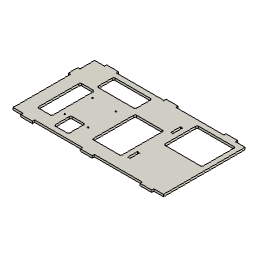
Base Plate (Autodesk Fusion 360 design; units mm, degrees)
Autodesk Fusion 360 part; units mm, degrees
sketch "Sketch1" plane through (0, 0, 0) normal (0, 0, 1) x (1, 0, 0)
  line L0 (160, -90) -> (-160, -90)
  line L1 (-160, -90) -> (-160, 90)
  line L2 (-160, 90) -> (160, 90)
  line L3 (160, 90) -> (160, -90)
  line L4 (160, -90) -> (-160, 90) construction
  line L5 (-160, -90) -> (160, 90) construction
  line L6 (170, 85.5) -> (-180, 85.5) construction
  line L7 (-180, -85.5) -> (170, -85.5) construction
  line L8 (-155.5, 90) -> (-155.5, -90)
  line L9 (-160, 90) -> (-135, 90)
  line L10 (-135, 90) -> (-135, 85.5)
  line L11 (-135, 85.5) -> (-160, 85.5)
  line L12 (-160, 85.5) -> (-160, 90)
  line L13 (-160, -90) -> (-135, -90)
  line L14 (-135, -90) -> (-135, -85.5)
  line L15 (-135, -85.5) -> (-160, -85.5)
  line L16 (-160, -85.5) -> (-160, -90)
  line L17 (-110, -90) -> (-10, -90)
  line L18 (-10, -90) -> (-10, -85.5)
  line L19 (-10, -85.5) -> (-110, -85.5)
  line L20 (-110, -85.5) -> (-110, -90)
  line L21 (-10, -90) -> (15, -90)
  line L22 (15, -90) -> (15, -85.5)
  line L23 (15, -85.5) -> (-10, -85.5)
  line L24 (-10, -85.5) -> (-10, -90)
  line L25 (15, -90) -> (115, -90)
  line L26 (115, -90) -> (115, -85.5)
  line L27 (115, -85.5) -> (15, -85.5)
  line L28 (15, -85.5) -> (15, -90)
  line L29 (115, -90) -> (140, -90)
  line L30 (140, -90) -> (140, -85.5)
  line L31 (140, -85.5) -> (115, -85.5)
  line L32 (115, -85.5) -> (115, -90)
  line L33 (-135, 85.5) -> (-110, 85.5)
  line L34 (-110, 85.5) -> (-110, 90)
  line L35 (-110, 90) -> (-135, 90)
  line L36 (-135, 90) -> (-135, 85.5)
  line L37 (-110, 85.5) -> (-10, 85.5)
  line L38 (-10, 85.5) -> (-10, 90)
  line L39 (-10, 90) -> (-110, 90)
  line L40 (-110, 90) -> (-110, 85.5)
  line L41 (-10, 85.5) -> (15, 85.5)
  line L42 (15, 85.5) -> (15, 90)
  line L43 (15, 90) -> (-10, 90)
  line L44 (-10, 90) -> (-10, 85.5)
  line L45 (15, 85.5) -> (115, 85.5)
  line L46 (115, 85.5) -> (115, 90)
  line L47 (115, 90) -> (15, 90)
  line L48 (15, 90) -> (15, 85.5)
  line L49 (115, 85.5) -> (140, 85.5)
  line L50 (140, 85.5) -> (140, 90)
  line L51 (140, 90) -> (115, 90)
  line L52 (115, 90) -> (115, 85.5)
  line L53 (140, 85.5) -> (160, 85.5)
  line L54 (160, 85.5) -> (160, 90)
  line L55 (160, 90) -> (140, 90)
  line L56 (140, 90) -> (140, 85.5)
  line L57 (140, -90) -> (160, -90)
  line L58 (160, -90) -> (160, -85.5)
  line L59 (160, -85.5) -> (140, -85.5)
  line L60 (140, -85.5) -> (140, -90)
  line L61 (-160, 55) -> (-155.5, 55)
  line L62 (-155.5, 55) -> (-155.5, 35)
  line L63 (-155.5, 35) -> (-160, 35)
  line L64 (-160, 35) -> (-160, 55)
  line L65 (-160, -35) -> (-155.5, -35)
  line L66 (-155.5, -35) -> (-155.5, -55)
  line L67 (-155.5, -55) -> (-160, -55)
  line L68 (-160, -55) -> (-160, -35)
  line L69 (55, 100) -> (55, -100) construction
  line L70 (59.5, 100) -> (59.5, -100) construction
  line L71 (55, 55) -> (59.5, 55)
  line L72 (59.5, 55) -> (59.5, 35)
  line L73 (59.5, 35) -> (55, 35)
  line L74 (55, 35) -> (55, 55)
  line L75 (55, -35) -> (59.5, -35)
  line L76 (59.5, -35) -> (59.5, -55)
  line L77 (59.5, -55) -> (55, -55)
  line L78 (55, -55) -> (55, -35)
  line L79 (-40.5, -43) -> (-89.5, -43) construction
  line L80 (-89.5, -43) -> (-89.5, 15) construction
  line L81 (-89.5, 15) -> (-40.5, 15) construction
  line L82 (-40.5, 15) -> (-40.5, -43) construction
  line L83 (-40.5, -43) -> (-89.5, 15) construction
  line L84 (-89.5, -43) -> (-40.5, 15) construction
  circle A0 centre (-40.5, 15) radius 1.4
  circle A1 centre (-89.5, 15) radius 1.4
  circle A2 centre (-89.5, -43) radius 1.4
  circle A3 centre (-40.5, -43) radius 1.4
  line L85 (-53, -75) -> (-77, -75)
  line L86 (-80, -72) -> (-80, -43)
  line L87 (-77, -40) -> (-53, -40)
  line L88 (-50, -43) -> (-50, -72)
  line L89 (-50, -75) -> (-80, -40) construction
  line L90 (-80, -75) -> (-50, -40) construction
  arc A4 (-77, -40) -> (-80, -43) centre (-77, -43) ccw
  arc A5 (-50, -43) -> (-53, -40) centre (-53, -43) ccw
  arc A6 (-80, -72) -> (-77, -75) centre (-77, -72) ccw
  arc A7 (-53, -75) -> (-50, -72) centre (-53, -72) ccw
  line L91 (-28, 40) -> (-102, 40)
  line L92 (-105, 43) -> (-105, 72)
  line L93 (-102, 75) -> (-28, 75)
  line L94 (-25, 72) -> (-25, 43)
  line L95 (-25, 40) -> (-105, 75) construction
  line L96 (-105, 40) -> (-25, 75) construction
  arc A8 (-102, 75) -> (-105, 72) centre (-102, 72) ccw
  arc A9 (-25, 72) -> (-28, 75) centre (-28, 72) ccw
  arc A10 (-105, 43) -> (-102, 40) centre (-102, 43) ccw
  arc A11 (-28, 40) -> (-25, 43) centre (-28, 43) ccw
  line L97 (147, 5) -> (73, 5)
  line L98 (70, 8) -> (70, 72)
  line L99 (73, 75) -> (147, 75)
  line L100 (150, 72) -> (150, 8)
  line L101 (150, 5) -> (70, 75) construction
  line L102 (70, 5) -> (150, 75) construction
  arc A12 (70, 8) -> (73, 5) centre (73, 8) ccw
  arc A13 (73, 75) -> (70, 72) centre (73, 72) ccw
  arc A14 (150, 72) -> (147, 75) centre (147, 72) ccw
  arc A15 (147, 5) -> (150, 8) centre (147, 8) ccw
  line L103 (42, -60) -> (-12, -60)
  line L104 (-15, -57) -> (-15, 27)
  line L105 (-12, 30) -> (42, 30)
  line L106 (45, 27) -> (45, -57)
  line L107 (45, -60) -> (-15, 30) construction
  line L108 (-15, -60) -> (45, 30) construction
  arc A16 (-12, 30) -> (-15, 27) centre (-12, 27) ccw
  arc A17 (45, 27) -> (42, 30) centre (42, 27) ccw
  arc A18 (-15, -57) -> (-12, -60) centre (-12, -57) ccw
  arc A19 (42, -60) -> (45, -57) centre (42, -57) ccw
  line L109 (-103, -60) -> (-127, -60)
  line L110 (-130, -57) -> (-130, 27)
  line L111 (-127, 30) -> (-103, 30)
  line L112 (-100, 27) -> (-100, -57)
  line L113 (-100, -60) -> (-130, 30) construction
  line L114 (-130, -60) -> (-100, 30) construction
  arc A20 (-127, 30) -> (-130, 27) centre (-127, 27) ccw
  arc A21 (-100, 27) -> (-103, 30) centre (-103, 27) ccw
  arc A22 (-130, -57) -> (-127, -60) centre (-127, -57) ccw
  arc A23 (-103, -60) -> (-100, -57) centre (-103, -57) ccw
  point P0 (-65, -14)
  point P1 (-65, -57.5)
  point P2 (-65, 57.5)
  point P3 (110, 40)
  point P4 (15, -15)
  point P5 (-115, -15)
  dimension "d1" = 320
  dimension "d2" = 180
  dimension "d3" = 4.5
  dimension "d4" = 4.5
  dimension "d5" = 4.5
  dimension "d6" = 25
  dimension "d7" = 25
  dimension "d8" = 100
  dimension "d9" = 25
  dimension "d10" = 25
  dimension "d11" = 100
  dimension "d12" = 25
  dimension "d13" = 25
  dimension "d14" = 100
  dimension "d15" = 25
  dimension "d16" = 100
  dimension "d17" = 25
  dimension "d18" = 20
  dimension "d19" = 20
  dimension "d20" = 35
  dimension "d21" = 35
  dimension "d22" = 215
  dimension "d23" = 4.5
  dimension "d24" = 20
  dimension "d25" = 20
  dimension "d26" = 35
  dimension "d27" = 35
  dimension "d28" = 49
  dimension "d29" = 58
  dimension "d30" = 76
  dimension "d31" = 120
  dimension "d32" = 2.8
  dimension "d33" = 2.8
  dimension "d34" = 2.8
  dimension "d35" = 2.8
  dimension "d46" = 30
  dimension "d47" = 35
  dimension "d48" = 3
  dimension "d49" = 3
  dimension "d50" = 3
  dimension "d51" = 3
  dimension "d52" = 80
  dimension "d53" = 35
  dimension "d54" = 25
  dimension "d55" = 3
  dimension "d56" = 3
  dimension "d57" = 3
  dimension "d58" = 3
  dimension "d65" = 80
  dimension "d66" = 70
  dimension "d67" = 3
  dimension "d68" = 3
  dimension "d69" = 3
  dimension "d70" = 3
  dimension "d71" = 3
  dimension "d72" = 3
  dimension "d73" = 3
  dimension "d74" = 3
  dimension "d75" = 3
  dimension "d76" = 3
  dimension "d77" = 3
  dimension "d78" = 3
  dimension "d103" = 10.5
  dimension "d104" = 10.5
  dimension "d105" = 10.5
  constraint horizontal L0
  constraint perpendicular L0 L1
  constraint parallel L0 L2
  constraint parallel L1 L3
  constraint coincident L4 origin
  constraint coincident L5 origin
  constraint perpendicular L3 L6
  constraint perpendicular L3 L7
  constraint perpendicular L0 L8
  constraint horizontal L9
  constraint vertical L10
  constraint horizontal L11
  constraint vertical L12
  constraint horizontal L13
  constraint vertical L14
  constraint horizontal L15
  constraint vertical L16
  constraint horizontal L17
  constraint vertical L18
  constraint horizontal L19
  constraint vertical L20
  constraint coincident L0 L17.start
  constraint horizontal L21
  constraint vertical L22
  constraint horizontal L23
  constraint vertical L24
  constraint horizontal L25
  constraint vertical L26
  constraint horizontal L27
  constraint vertical L28
  constraint horizontal L29
  constraint vertical L30
  constraint horizontal L31
  constraint vertical L32
  constraint horizontal L33
  constraint vertical L34
  constraint horizontal L35
  constraint vertical L36
  constraint horizontal L37
  constraint vertical L38
  constraint horizontal L39
  constraint vertical L40
  constraint horizontal L41
  constraint vertical L42
  constraint horizontal L43
  constraint vertical L44
  constraint horizontal L45
  constraint vertical L46
  constraint horizontal L47
  constraint vertical L48
  constraint horizontal L49
  constraint vertical L50
  constraint horizontal L51
  constraint vertical L52
  constraint horizontal L53
  constraint vertical L54
  constraint horizontal L55
  constraint vertical L56
  constraint horizontal L57
  constraint vertical L58
  constraint horizontal L59
  constraint vertical L60
  constraint coincident L3 L58.end
  constraint coincident L7 L58.end
  constraint horizontal L61
  constraint vertical L62
  constraint horizontal L63
  constraint vertical L64
  constraint coincident L1 L61.start
  constraint horizontal L65
  constraint vertical L66
  constraint horizontal L67
  constraint vertical L68
  constraint coincident L1 L65.start
  constraint coincident L2 L8.start
  constraint perpendicular L47 L69
  constraint perpendicular L25 L70
  constraint horizontal L71
  constraint vertical L72
  constraint horizontal L73
  constraint vertical L74
  constraint coincident L69 L71.start
  constraint horizontal L75
  constraint vertical L76
  constraint horizontal L77
  constraint vertical L78
  constraint coincident L69 L75.start
  constraint horizontal L79
  constraint perpendicular L79 L80
  constraint parallel L79 L81
  constraint parallel L80 L82
  constraint coincident L83 P0
  constraint coincident L84 P0
  constraint coincident L81.end L82.start
  constraint coincident L80.end L81.start
  constraint coincident L79.end L80.start
  constraint coincident L79.start L82.end
  constraint horizontal L85
  constraint perpendicular L85 L86
  constraint parallel L85 L87
  constraint parallel L86 L88
  constraint coincident L89 P1
  constraint coincident L90 P1
  constraint coincident L89.end L87
  constraint coincident L89.end L86
  constraint tangent L87 A4
  constraint tangent L86 A4
  constraint coincident L90.end L87
  constraint coincident L90.end L88
  constraint tangent L87 A5
  constraint tangent L88 A5
  constraint coincident L90.start L86
  constraint coincident L90.start L85
  constraint tangent L86 A6
  constraint tangent L85 A6
  constraint coincident L89.start L85
  constraint coincident L89.start L88
  constraint tangent L85 A7
  constraint tangent L88 A7
  constraint horizontal L91
  constraint perpendicular L91 L92
  constraint parallel L91 L93
  constraint parallel L92 L94
  constraint coincident L95 P2
  constraint coincident L96 P2
  constraint coincident L95.end L92
  constraint coincident L95.end L93
  constraint tangent L92 A8
  constraint tangent L93 A8
  constraint coincident L96.end L93
  constraint coincident L96.end L94
  constraint tangent L93 A9
  constraint tangent L94 A9
  constraint coincident L96.start L92
  constraint coincident L96.start L91
  constraint tangent L92 A10
  constraint tangent L91 A10
  constraint coincident L95.start L91
  constraint coincident L95.start L94
  constraint tangent L91 A11
  constraint tangent L94 A11
  constraint vertical P0 P2
  constraint vertical P0 P1
  constraint horizontal L97
  constraint perpendicular L97 L98
  constraint parallel L97 L99
  constraint parallel L98 L100
  constraint coincident L101 P3
  constraint coincident L102 P3
  constraint coincident L102.start L97
  constraint coincident L102.start L98
  constraint tangent L97 A12
  constraint tangent L98 A12
  constraint coincident L101.end L98
  constraint coincident L101.end L99
  constraint tangent L98 A13
  constraint tangent L99 A13
  constraint coincident L102.end L99
  constraint coincident L102.end L100
  constraint tangent L99 A14
  constraint tangent L100 A14
  constraint coincident L101.start L97
  constraint coincident L101.start L100
  constraint tangent L97 A15
  constraint tangent L100 A15
  constraint horizontal L103
  constraint perpendicular L103 L104
  constraint parallel L103 L105
  constraint parallel L104 L106
  constraint coincident L107 P4
  constraint coincident L108 P4
  constraint coincident L107.end L104
  constraint coincident L107.end L105
  constraint tangent L104 A16
  constraint tangent L105 A16
  constraint coincident L108.end L105
  constraint coincident L108.end L106
  constraint tangent L105 A17
  constraint tangent L106 A17
  constraint coincident L108.start L104
  constraint coincident L108.start L103
  constraint tangent L104 A18
  constraint tangent L103 A18
  constraint coincident L107.start L103
  constraint coincident L107.start L106
  constraint tangent L103 A19
  constraint tangent L106 A19
  constraint horizontal L109
  constraint perpendicular L109 L110
  constraint parallel L109 L111
  constraint parallel L110 L112
  constraint coincident L113 P5
  constraint coincident L114 P5
  constraint coincident L113.end L110
  constraint coincident L113.end L111
  constraint tangent L110 A20
  constraint tangent L111 A20
  constraint coincident L114.end L111
  constraint coincident L114.end L112
  constraint tangent L111 A21
  constraint tangent L112 A21
  constraint coincident L114.start L110
  constraint coincident L114.start L109
  constraint tangent L110 A22
  constraint tangent L109 A22
  constraint coincident L113.start L109
  constraint coincident L113.start L112
  constraint tangent L109 A23
  constraint tangent L112 A23
  measures "d1" distance of L1.end L2.end
  measures "d2" distance of L0.end L1.end
  measures "d3" distance of L0 L7
  measures "d4" distance of L2 L6
  measures "d5" distance of L1 L8
  measures "d6" distance of L1.end L9.end
  measures "d7" distance of L0.end L13.end
  measures "d8" distance of L17.start L17.end
  measures "d9" distance of L14 L20
  measures "d10" distance of L17.end L21.end
  measures "d11" distance of L21.end L25.end
  measures "d12" distance of L25.end L29.end
  measures "d13" distance of L10.end L33.end
  measures "d14" distance of L33.end L37.end
  measures "d15" distance of L37.end L41.end
  measures "d16" distance of L41.end L45.end
  measures "d17" distance of L45.end L49.end
  measures "d18" distance of L61.start L63.end
  measures "d19" distance of L65.start L67.end
  measures "d20" distance of L13 L67
  measures "d21" distance of L9 L61
  measures "d22" distance of L1 L69
  measures "d23" distance of L69 L70
  measures "d24" distance of L71.start L73.end
  measures "d25" distance of L75.start L77.end
  measures "d26" distance of L25 L77
  measures "d27" distance of L2 L71
  measures "d28" distance of L80.end L81.end
  measures "d29" distance of L79.end L80.end
  measures "d30" distance of L0 P0
  measures "d31" distance of L69 P0
  measures "d32" diameter of A0
  measures "d33" diameter of A1
  measures "d34" diameter of A2
  measures "d35" diameter of A3
  measures "d46" distance of L89.end L90.end
  measures "d47" distance of L90.start L89.end
  measures "d48" radius of A4
  measures "d49" radius of A5
  measures "d50" radius of A6
  measures "d51" radius of A7
  measures "d52" distance of L95.end L96.end
  measures "d53" distance of L96.start L95.end
  measures "d54" distance of L81.end L91
  measures "d55" radius of A8
  measures "d56" radius of A9
  measures "d57" radius of A10
  measures "d58" radius of A11
  measures "d65" distance of L101.start L102.start
  measures "d66" distance of L101.start L102.end
  measures "d67" radius of A12
  measures "d68" radius of A13
  measures "d69" radius of A14
  measures "d70" radius of A15
  measures "d71" radius of A16
  measures "d72" radius of A17
  measures "d73" radius of A18
  measures "d74" radius of A19
  measures "d75" radius of A20
  measures "d76" radius of A21
  measures "d77" radius of A22
  measures "d78" radius of A23
  measures "d103" distance of L19 L85
  measures "d104" distance of L37 L93
  measures "d105" distance of L6 L99
extrude "Extrude1" add sketch "Sketch1" along normal blind 4.5 contours L0 L26 L29 L30 L31 L32 L60 | L0 L3 L8 L11 L14 L15 L19 L20 L23 L27 L31 L33 L37 L41 L45 L49 L53 L59 L62 L66 | L0 L18 L21 L22 L23 L24 L28 | L2 L46 L49 L50 L51 L52 L56 | L2 L38 L41 L42 L43 L44 L48 | L2 L10 L33 L34 L35 L36 L40 | L1 L8 L61 L62 L63 L64
move_face "OffsetFaces1" offset -0.1 6 faces at (140, -88.5, 1.5) (15, -88.5, 1.5) (-110, -87, 1.5) (140, 87, 1.5) (15, 87, 1.5) (-110, 87, 1.5)
move_face "OffsetFaces2" offset -0.1 6 faces at (115, -88.5, 1.5) (-10, -88.5, 1.5) (-135, -88.5, 3) (-135, 88.5, 1.5) (-10, 87, 1.5) (115, 87, 1.5)
move_face "OffsetFaces5" offset -0.1 1 faces at (-157, 35, 1.5)
move_face "OffsetFaces6" offset -0.1 1 faces at (-158.5, 55, 1.5)
